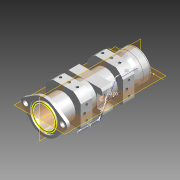
# Autodesk Inventor part: 01104
Saved by Autodesk Inventor 2015 (Build 190159000, 159)
## iProperties
Created: 2015-04-14
Part Number: 01104
Material: Aluminum 6061
Description: Main throttle body
Document SubType Name: Modeling
Designer: FC
Density: 2.7 g/cm^3
Appearance: Aluminum - Flat
Part Category: 5 - Engine
Author: FC
Autodesk Inventor part; units mm, degrees
ref_plane "XZ Plane" through (0, 0, 0) normal (0, 1, 0) x (-1, 0, 0)
sketch "Sketch1" plane through (0, 0, 0) normal (0, 0, 1) x (1, 0, 0)
  line L0 (14, -120) -> (14, -22.588)
  line L1 (14.382, -20.4813) -> (16.618, -14.5187)
  line L2 (17, -12.412) -> (17, -2)
  line L3 (19, -13.8627) -> (16, -21.8627)
  line L4 (16, -21.8627) -> (16, -120)
  line L5 (19.5, 0) -> (19, 0)
  line L6 (16, -120) -> (14, -120)
  line L7 (19, -1) -> (19.4, -1)
  line L8 (19.4, -1) -> (19.4, 0)
  line L9 (19.4, 0) -> (19.5, 0)
  line L10 (19, -8.5) -> (19.4, -8.5)
  line L11 (19.4, -8.5) -> (19.4, -9.5)
  line L12 (19.4, -9.5) -> (19, -9.5)
  line L13 (19, -9.5) -> (19, -13.8627)
  line L14 (19, -1) -> (19, -8.5)
  line L15 (0, 0) -> (0, -57.1164)
  arc A0 (19, 0) -> (17, -2) centre (19, -2) ccw
  line L16 (-23.8, 0) -> (30.8, 0) construction
  line L17 (14, -21.5) -> (14.382, -20.4813)
  line L18 (14, -22.588) -> (14, -21.5)
  line L19 (16.618, -14.5187) -> (17, -13.5)
  line L20 (17, -12.412) -> (17, -13.5)
  point P0 (17, 0)
  point P1 (17, 0)
  point P2 (16, -38.699)
  dimension "d1" = 13.5
  dimension "d2" = 21.5
  dimension "d3" = 14
  dimension "d4" = 120
  dimension "d5" = 2
  dimension "d6" = 0.4
  dimension "d7" = 1
  dimension "d8" = 0.4
  dimension "d9" = 1
  dimension "d10" = 8.5
  dimension "d124" = 19
  dimension "d125" = 2
  dimension "d126" = 2
  dimension "d127" = 2
  constraints: 40 end point, 8 point on line, 5 parallel, 3 collinear, 3 vertical, 2 coincident, 2 horizontal, 2 perpendicular, 2 point on circle, 2 tangent, 1 centre point, 1 other
  measures "d1" distance of L19.end point (17, 0)
  measures "d2" vertical distance of L17.start point (17, 0)
  measures "d3" distance from line of L15.start L0
  measures "d4" vertical distance of point (17, 0) L0.start
  measures "d5" distance between parallel lines of L1 L3
  measures "d6" distance of L7.start L7.end
  measures "d7" distance of L7.end L8.end
  measures "d8" distance of L11.end L12.end
  measures "d9" distance of L10.end L11.end
  measures "d10" distance between parallel lines of L9 L10
  measures "d124" distance between parallel lines of L15 L14
  measures "d125" distance between parallel lines of L2 L14
  measures "d126" distance from line of L2 L12.end
  measures "d127" radius of A0
revolve "Revolution1" add sketch "Sketch1" angle 360 about axis through (0, 0, 0) along (0, -1, 0)
sketch "Sketch5" plane through (0, -120, 0) normal (0, -1, 0) x (1, 0, 0)
  circle A0 centre (0, 0) radius 14 projected
  circle A1 centre (0, 0) radius 16 projected
  point P0 (-16, 0)
  constraints: 1 horizontal alignment, 1 other
sketch "Sketch7" plane through (0, -120, 0) normal (0, -1, 0) x (1, 0, 0)
  circle A0 centre (0, 0) radius 14 projected
  circle A1 centre (-24, 3.5) radius 3.25
  circle A2 centre (24, 3.5) radius 3.25
  circle A3 centre (0, 0) radius 18.5
  line L0 (-34.5214, 0) -> (40.2242, 0) construction
  circle A4 centre (0, 0) radius 14 construction
  line L1 (0, -32.9352) -> (0, 39.8381)
  arc A5 (-27.266, 8.5332) -> (-28.5674, -0.3909) centre (-24, 3.5) ccw
  arc A6 (28.5674, -0.3909) -> (27.266, 8.5332) centre (24, 3.5) ccw
  arc A7 (-16.7472, -14.2665) -> (16.7472, -14.2665) centre (0, 0) ccw
  arc A8 (11.9753, 18.4551) -> (-11.9753, 18.4551) centre (0, 0) ccw
  line L2 (-11.9753, 18.4551) -> (-27.266, 8.5332)
  line L3 (11.9753, 18.4551) -> (27.266, 8.5332)
  line L4 (28.5674, -0.3909) -> (16.7472, -14.2665)
  line L5 (-16.7472, -14.2665) -> (-28.5674, -0.3909)
  point P0 (0, -18.5)
  dimension "d28" = 37
  dimension "d24" = 6.5
  dimension "d27" = 6.5
  dimension "d148" = 3.5
  dimension "d149" = 22
  dimension "d150" = 6
  dimension "d151" = 6
  dimension "d152" = 3.5
  dimension "d155" = 48
  dimension "d157" = 24
  constraints: 12 end point, 9 point on circle, 8 tangent, 6 centre point, 4 coincident, 2 point on line, 1 horizontal, 1 vertical, 1 vertical alignment, 3 other
  measures "d24" diameter of A2
  measures "d27" diameter of A1
  measures "d148" distance from line of L0 A1.centre
  measures "d149" radius of A8
  measures "d150" radius of A5
  measures "d151" radius of A6
  measures "d152" distance from line of L0 A2.centre
  measures "d155" distance of A1.centre A2.centre
  measures "d157" horizontal distance of A2.centre point (0, 0)
extrude "Extrusion2" add sketch "Sketch7" against normal blind 4 contours A0 L1 A3 | A0 L1 A3 | L1 A8 L3 A6 L4 A7 A3 | A3 L1 A7 L5 A5 L2 A8
sketch "Sketch8" plane through (0, -120, 9.4936) normal (0, -1, 0) x (1, 0, 0)
  circle A0 centre (0, -9.4936) radius 16
  circle A1 centre (0, -9.4936) radius 18.5 projected
  circle A2 centre (0, -9.4936) radius 18.5
  constraints: 2 centre point, 2 coincident, 1 concentric
extrude "Extrusion3" cut sketch "Sketch8" against normal blind 2
fillet "Fillet1" radius 2 1 edges at (-16, -116, 0)
sketch "Sketch9" plane through (0, 0, 0) normal (1, 0, 0) x (0, 1, 0)
  line L0 (-21.8627, 16) -> (-114, 16) projected
  line L1 (-21.8627, 16) -> (-21.8627, -16) projected
  line L2 (-32.5282, 0) -> (-141.2862, 0) construction
  line L3 (-53, -16) -> (-67, -16)
  line L4 (-67, -16) -> (-67, -26.5)
  line L5 (-67, -26.5) -> (-53, -26.5)
  line L6 (-53, -26.5) -> (-53, -16)
  line L7 (-80, -16) -> (-95, -16)
  line L8 (-95, -16) -> (-95, -26.5)
  line L9 (-95, -26.5) -> (-80, -26.5)
  line L10 (-80, -26.5) -> (-80, -16)
  line L11 (-21.8627, -16) -> (-114, -16) construction
  line L12 (-40, -16) -> (-25, -16)
  line L13 (-25, -16) -> (-25, -26.5)
  line L14 (-25, -26.5) -> (-40, -26.5)
  line L15 (-40, -26.5) -> (-40, -16)
  line L16 (-87.5, -26.5) -> (-87.5, -22.6244) construction
  line L17 (-60, -26.5) -> (-60, -20.6547) construction
  line L18 (0, 19.4) -> (0, -19.4) projected
  point P0 (0, 0)
  dimension "d42" = 14
  dimension "d47" = 10.5
  dimension "d55" = 10.5
  dimension "d57" = 35
  dimension "d58" = 20
  dimension "d59" = 20
  dimension "d60" = 35
  dimension "d61" = 10.5
  dimension "d147" = 60
  constraints: 30 end point, 6 parallel, 4 horizontal, 3 perpendicular, 2 collinear, 2 midpoint, 2 vertical, 1 point on line
  measures "d42" distance of L4.end L5.end
  measures "d47" distance of L5.end L3.start
  measures "d55" distance of L9.end L7.start
  measures "d57" distance between parallel lines of L8 L17
  measures "d58" distance between parallel lines of L10 L17
  measures "d59" distance between parallel lines of L15 L17
  measures "d60" distance between parallel lines of L13 L17
  measures "d61" distance of L12.end L13.end
  measures "d147" distance from line of L17.start L18
revolve "Revolution2" add sketch "Sketch9" angle 360 about axis through (0, -32.5282, 0) along (0, -1, 0)
sketch "Sketch10" plane through (0, 0, 0) normal (1, 0, 0) x (0, 1, 0)
  line L0 (-95, 16) -> (-114, 16) construction
  line L1 (-95, -16) -> (-114, -16) construction
  line L2 (-53, 26.5) -> (-53, -26.5) construction
  line L3 (-67, 26.5) -> (-67, -26.5) construction
  circle A0 centre (-60, 0) radius 4
  line L4 (-53, -26.5) -> (-67, -26.5) projected
  line L5 (-144, 0) -> (24, 0) construction
  point P0 (0, 0)
  point P1 (-60, -26.5)
  dimension "d50" = 8
  constraints: 2 midpoint, 1 centre point, 1 vertical alignment
  measures "d50" diameter of A0
extrude "Extrusion4" cut sketch "Sketch10" along normal through all both and the other way through all
sketch "Sketch11" plane through (0, 0, 0) normal (0, 0, 1) x (1, 0, 0)
  line L0 (-26.5, -53) -> (26.5, -53) construction
  line L1 (16, -53) -> (-16, -53) construction
  line L2 (-26.5, -53) -> (26.5, -53) construction
  line L3 (14, -120) -> (14, -21.5) construction
  line L4 (14, -120) -> (14, -21.5) construction
  line L5 (14, -120) -> (14, -21.5) construction
  line L6 (14, -120) -> (14, -21.5) construction
  line L7 (-14, -120) -> (-14, -21.5) construction
  line L8 (-26.5, -53) -> (-26.5, -67) construction
  line L9 (-26.5, -67) -> (26.5, -67) construction
  line L10 (27.5381, -60) -> (-34.1758, -60)
  line L11 (16, -40) -> (16, -53) construction
  line L12 (-16, -40) -> (-16, -53) construction
  line L13 (-16, -67) -> (-16, -80) construction
  line L14 (16, -67) -> (16, -80) construction
  line L15 (26.5, -53) -> (26.5, -67) construction
  line L16 (26.5, -60) -> (16, -60)
  line L17 (16, -60) -> (16, -49)
  line L18 (16, -49) -> (26.5, -49)
  line L19 (26.5, -49) -> (26.5, -60)
  line L20 (-26.5, -60) -> (-16, -60)
  line L21 (-16, -60) -> (-16, -49)
  line L22 (-16, -49) -> (-26.5, -49)
  line L23 (-26.5, -49) -> (-26.5, -60)
  line L24 (-19.6, -60) -> (19.6, -60) construction
  point P0 (0, 0)
  dimension "d62" = 11
  constraints: 20 end point, 4 horizontal, 4 parallel, 4 point on line, 2 midpoint, 2 perpendicular, 1 collinear, 2 other
  measures "d62" distance of L22.end L20.start
revolve "Revolution3" cut sketch "Sketch11" angle 360 about axis through (27.5381, -60, 0) along (-1, 0, 0)
sketch "Sketch12" plane through (0, 0, 0) normal (0, 0, 1) x (1, 0, 0)
  line L0 (-25.1048, -53) -> (25.1048, -53) construction
  line L1 (-25.1048, -67) -> (25.1048, -67) construction
  line L2 (-16, -40) -> (-16, -53) construction
  line L3 (-16, -67) -> (-16, -80) construction
  line L4 (16, -40) -> (16, -53) construction
  line L5 (16, -67) -> (16, -80) construction
  line L6 (-25.1048, -53) -> (-23, -53)
  line L7 (-23, -53) -> (-23, -67)
  line L8 (-23, -67) -> (-25.1048, -67)
  line L9 (-25.1048, -67) -> (-25.1048, -53)
  line L10 (-25.1048, -67) -> (-16, -67) construction
  line L11 (0, 4.0598) -> (0, -79.7186) construction
  line L12 (25.1048, -53) -> (23, -53)
  line L13 (23, -53) -> (23, -67)
  line L14 (23, -67) -> (25.1048, -67)
  line L15 (25.1048, -67) -> (25.1048, -53)
  line L16 (-26.5, -25) -> (-26.5, -40) construction
  line L17 (-26.5, -25) -> (26.5, -25) construction
  line L18 (-25.1048, -53) -> (25.1048, -53) construction
  line L19 (-26.5, -80) -> (26.5, -80) construction
  line L20 (-26.5, -95) -> (26.5, -95) construction
  line L21 (-26.5, -40) -> (26.5, -40) construction
  line L22 (-26.5, -40) -> (-23, -40)
  line L23 (-23, -40) -> (-23, -25)
  line L24 (-23, -25) -> (-26.5, -25)
  line L25 (-26.5, -25) -> (-26.5, -40)
  line L26 (-26.5, -80) -> (-23, -80)
  line L27 (-23, -80) -> (-23, -95)
  line L28 (-23, -95) -> (-26.5, -95)
  line L29 (-26.5, -95) -> (-26.5, -80)
  line L30 (-16, -21.8627) -> (-16, -25) construction
  line L31 (-16, -95) -> (-16, -114) construction
  line L32 (26.5, -25) -> (26.5, -40) construction
  line L33 (26.5, -40) -> (23, -40)
  line L34 (23, -40) -> (23, -25)
  line L35 (23, -25) -> (26.5, -25)
  line L36 (26.5, -25) -> (26.5, -40)
  line L37 (26.5, -80) -> (23, -80)
  line L38 (23, -80) -> (23, -95)
  line L39 (23, -95) -> (26.5, -95)
  line L40 (26.5, -95) -> (26.5, -80)
  point P0 (0, 0)
  point P1 (25.1048, -53)
  point P2 (25.1048, -67)
  dimension "d64" = 7
  dimension "d69" = 7
  constraints: 52 end point, 14 symmetric about line, 6 parallel, 6 point on line, 3 horizontal, 3 perpendicular, 1 vertical
  measures "d64" distance between parallel lines of L2 L7
  measures "d69" distance between parallel lines of L30 L23
extrude "Extrusion5" cut sketch "Sketch12" along normal through all both and the other way through all
sketch "Sketch13" plane through (0, 0, 0) normal (1, 0, 0) x (0, 1, 0)
  line L0 (-25, 26.5) -> (-25, -26.5) construction
  line L1 (-40, 16) -> (-53, 16) construction
  line L2 (-33.4184, 0) -> (-136.7664, 0) construction
  line L3 (-80, -26.5) -> (-95, -26.5) construction
  line L4 (-25, -26.5) -> (-40, -26.5) construction
  line L5 (-53, -26.5) -> (-67, -26.5) construction
  line L6 (-40, -16) -> (-53, -16) construction
  line L7 (-25, -26.5) -> (-95, -26.5)
  line L8 (-95, -26.5) -> (-95, -16)
  line L9 (-95, -16) -> (-25, -16)
  line L10 (-25, -16) -> (-25, -26.5)
  line L11 (-40, 16) -> (-40, -16) projected
  line L12 (-53, 26.5) -> (-67, 26.5)
  line L13 (-67, 26.5) -> (-67, 16)
  line L14 (-67, 16) -> (-53, 16)
  line L15 (-53, 16) -> (-53, 26.5)
  line L16 (-40, 26.5) -> (-40, 13.1624) projected
  line L17 (-25, 26.5) -> (-40, 26.5)
  line L18 (-40, 26.5) -> (-40, 23)
  line L19 (-40, 23) -> (-25, 23)
  line L20 (-25, 23) -> (-25, 26.5)
  line L21 (-95, 26.5) -> (-95, 13.1624) projected
  line L22 (-80, 26.5) -> (-95, 26.5)
  line L23 (-95, 26.5) -> (-95, 23)
  line L24 (-95, 23) -> (-80, 23)
  line L25 (-80, 23) -> (-80, 26.5)
  point P0 (0, 0)
  point P1 (-95, 26.5)
  point P2 (-67, 26.5)
  point P3 (-95, 16)
  point P4 (-95, -16)
  point P5 (-80.9184, 16)
  dimension "d113" = 7
  constraints: 42 end point, 11 symmetric about line, 6 parallel, 4 horizontal, 3 perpendicular, 3 point on line
  measures "d113" distance between parallel lines of L1 L19
extrude "Extrusion6" cut sketch "Sketch13" along normal through all both and the other way through all
sketch "Sketch14" plane through (-23, -40, 13.1624) normal (-1, 0, 0) x (0, 0, 1)
  line L0 (-13.1624, 64.9184) -> (-13.1624, -103.0816) construction
  line L1 (-26.3249, 15) -> (0, 15) construction
  line L2 (0, -40) -> (0, -55) construction
  line L3 (-26.3249, -40) -> (0, -40) construction
  line L4 (-26.3249, -55) -> (-26.3249, -40) construction
  line L5 (0, -55) -> (-26.3249, -55) construction
  circle A0 centre (-22.1624, 7.5) radius 2 construction
  circle A1 centre (-22.1624, -47.5) radius 2 construction
  line L6 (-26.3249, 0) -> (-26.3249, 15) construction
  line L7 (-26.3249, -55) -> (-26.3249, -40) construction
  line L8 (-13.1624, 17.742) -> (-13.1624, -35.3687)
  circle A2 centre (-4.1624, 7.5) radius 2 construction
  circle A3 centre (-4.1624, -47.5) radius 2 construction
  point P0 (-13.1624, 40)
  point P1 (-26.3249, 7.5)
  point P2 (-26.3249, -47.5)
  point P3 (-26.3249, -47.5)
  point P4 (-26.3249, 7.5)
  dimension "d86" = 4
  dimension "d87" = 4
  dimension "d88" = 9
  dimension "d89" = 9
  constraints: 4 centre point, 4 end point, 4 midpoint, 2 horizontal alignment, 2 point on line, 2 symmetric about line, 2 other
  measures "d86" diameter of A0
  measures "d87" diameter of A1
  measures "d88" distance from line of L0 A1.centre
  measures "d89" distance from line of L0 A0.centre
hole "Hole4" at (-23, -32.5, -9) at (-23, -87.5, -9) at (-23, -32.5, 9) at (-23, -87.5, 9) direction (1, 0, 0) diameter 3.242 depth 6 tip angle 118 thread size "M4x0.7" class "6H" standard "ISO Metric profile"
sketch "Sketch15" plane through (-23, -40, 13.1624) normal (-1, 0, 0) x (0, 0, 1)
  circle A0 centre (-13.1624, 10.5) radius 2.25 projected
  circle A1 centre (-13.1624, -44.5) radius 2.25 projected
  point P0 (-13.1624, 40)
hole "Hole5" at (-23, -29.5, 0) at (-23, -84.5, 0) direction (1, 0, 0) diameter 4.134 depth 7 tip angle 118 thread size "M5x0.8" class "6H" standard "ISO Metric profile"
sketch "Sketch16" plane through (23, -40, -13.1624) normal (1, 0, 0) x (0, 0, -1)
  circle A0 centre (-13.1624, 4.5) radius 2.25 projected
  circle A1 centre (-13.1624, -50.5) radius 2.25 projected
  point P0 (-13.1624, 40)
hole "Hole6" at (23, -35.5, 0) at (23, -90.5, 0) direction (-1, 0, 0) diameter 4.134 depth 7 tip angle 118 thread size "M5x0.8" class "6H" standard "ISO Metric profile"
sketch "Sketch17" plane through (23, -40, -13.1624) normal (1, 0, 0) x (0, 0, -1)
  line L0 (-13.1624, -20) -> (-30.483, -10) construction
  line L1 (-13.1624, -37.5) -> (-13.1624, -2.5) construction
  line L2 (-30.483, -10) -> (-30.483, 19) construction
  line L3 (-13.1624, -20) -> (4.1581, -30) construction
  line L4 (2.8376, -55) -> (2.8376, -40) construction
  line L5 (4.1581, -30) -> (4.1581, -59) construction
  point P0 (-13.1624, 40)
  dimension "d118" = 20
  dimension "d119" = 60
  dimension "d120" = 29
  dimension "d121" = 20
  dimension "d123" = 29
  constraints: 10 end point, 3 vertical, 1 collinear, 3 other
  measures "d118" distance of L0.start L0.end
  measures "d119" angle of L1 L0
  measures "d120" distance of L0.end L2.end
  measures "d121" distance of L0.start L3.end
  measures "d123" distance of L3.end L5.end
mirror "Mirror1" about plane through (0, 0, 0) normal (1, 0, 0) of "Hole4"
sketch "Sketch18" plane through (-13.1624, -40, 23) normal (0, 0, 1) x (1, 0, 0)
  line L0 (0, 0) -> (0, 15) construction
  line L1 (26.3249, 0) -> (0, 0) construction
  line L2 (26.3249, 15) -> (26.3249, 0) construction
  line L3 (0, 15) -> (26.3249, 15) construction
  line L4 (0, -55) -> (0, -40) construction
  line L5 (26.3249, -55) -> (0, -55) construction
  line L6 (26.3249, -40) -> (26.3249, -55) construction
  line L7 (0, -40) -> (26.3249, -40) construction
  line L8 (13.1624, -104) -> (13.1624, 64) construction
  point P0 (13.1624, 40)
  point P1 (13.1624, 7.5)
  point P2 (13.1624, -47.5)
  constraints: 2 point on line
hole "Hole7" at (0, -32.5, 23) at (0, -87.5, 23) direction (0, 0, -1) diameter 4 depth 23 tip angle 118
sketch "Sketch19" plane through (-13.1624, -40, 23) normal (0, 0, 1) x (1, 0, 0)
  circle A0 centre (13.1624, 7.5) radius 2 construction
  line L0 (0, 0) -> (0, 15) construction
  line L1 (26.3249, 0) -> (0, 0) construction
  line L2 (26.3249, 15) -> (26.3249, 0) construction
  line L3 (0, 15) -> (26.3249, 15) construction
  circle A1 centre (13.1624, -47.5) radius 2 construction
  line L4 (0, -55) -> (0, -40) construction
  line L5 (26.3249, -55) -> (0, -55) construction
  line L6 (26.3249, -40) -> (26.3249, -55) construction
  line L7 (0, -40) -> (26.3249, -40) construction
  line L8 (13.1624, 22.1397) -> (13.1624, -67.6131) construction
  line L9 (13.1624, 7.5) -> (24.1624, 7.5) construction
  line L10 (13.1624, 7.5) -> (2.1624, 7.5) construction
  line L11 (13.1624, -47.5) -> (2.1624, -47.5) construction
  line L12 (13.1624, -47.5) -> (24.1624, -47.5) construction
  point P0 (13.1624, 40)
  dimension "d144" = 22
  dimension "d145" = 22
  dimension "d146" = 0
  constraints: 10 end point, 2 horizontal, 1 collinear, 1 perpendicular, 1 symmetric about line, 1 vertical, 1 vertical alignment
  measures "d144" diameter of L9.end L8
  measures "d145" distance of L11.end L12.end
  measures "d146" distance from line of L11.start L8
hole "Hole8" at (-11, -32.5, 23) at (11, -32.5, 23) at (11, -87.5, 23) at (-11, -87.5, 23) direction (0, 0, -1) diameter 3.242 depth 6 tip angle 118 thread size "M4x0.7" class "6H" standard "ISO Metric profile"
equation "\"d53\" = d50"
body "Solid1"
